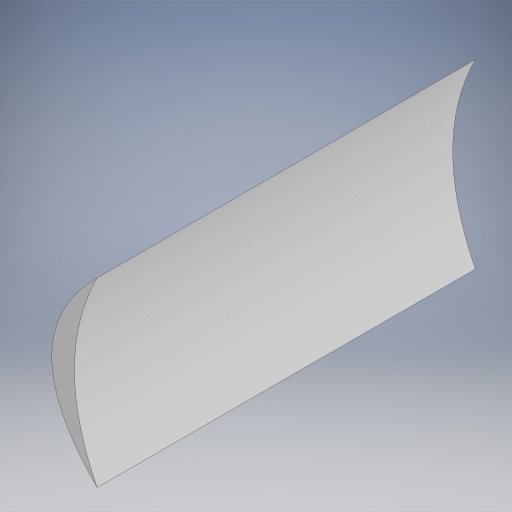
# Autodesk Inventor part: CE-2.1.2
Saved by Autodesk Inventor 2024 (Build 280153000, 153)
## iProperties
Created: 2024-01-31
Part Number: CE-2.1.2
Material: Generic
Document SubType Name: Modeling
Designer: Alex
Density: 1 g/cm^3
Appearance: Default
Author: Alex
Autodesk Inventor part; units mm, degrees
ref_plane "YZ Plane" through (0, 0, 0) normal (1, 0, 0) x (0, 1, 0)
ref_plane "XZ Plane" through (0, 0, 0) normal (0, 1, 0) x (-1, 0, 0)
ref_plane "XY Plane" through (0, 0, 0) normal (0, 0, 1) x (1, 0, 0)
sketch "Sketch1" plane through (0, 0, 0) normal (0, 0, 1) x (1, 0, 0)
  spline S0 degree 5 poles (3, -6) (2.3135, -5.3143) (1.6789, -4.5783) (1.1054, -3.7875) (0.2499, -2.192) (-0.0709, -0.4172) (-0.0709, 0.4172) (0.2499, 2.192) (1.1054, 3.7875) (1.6789, 4.5783) (2.3135, 5.3143) (3, 6) knots 0 0 0 0 0 0 0.352148 0.352148 0.352148 0.647852 0.647852 0.647852 1 1 1 1 1 1
  spline S1 degree 4 poles (3, -6) (2.3035, -4.6049) (1.7732, -3.1213) (1.2264, 0) (1.7732, 3.1213) (2.3035, 4.6049) (3, 6) knots 0 0 0 0 0 0.5 0.5 1 1 1 1 1
  point P0 (0, 0)
  dimension "d4" = 6
  dimension "d5" = 3
  dimension "d6" = 6
  constraints: 2 vertical alignment, 4 other
  measures "d4" vertical distance of point (0, 0) point (3, 6)
  measures "d5" horizontal distance of point (0, 0) point (3, -6)
  measures "d6" vertical distance of point (0, 0) point (3, -6)
extrude "Extrusion1" add sketch "Sketch1" along normal mid plane 25
equation "curve S0 of \"Sketch1\": x = ( 1 mm * (t^2) ) / (12 mm); y = 1 mm * t; t from d0 to d1"
equation "curve S1 of \"Sketch1\": x = ( ( 1 mm * t^2) + 36 mm) / 24 mm; y = 1 mm * t; t from d2 to d3"
body "Solid1"
